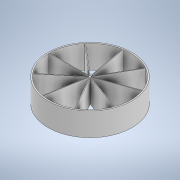
# Autodesk Inventor part: Деталь1
Saved by Autodesk Inventor 2022 (Build 260153000, 153)
## iProperties
Created: 2023-03-14
Part Number: Деталь1
Material: Типовые
Document SubType Name: Modeling
Designer: lrnto01
Density: 1 g/cm^3
Appearance: По умолчанию
Author: lrnto01
Autodesk Inventor part; units mm, degrees
ref_plane "YZ Plane" through (0, 0, 0) normal (1, 0, 0) x (0, 1, 0)
ref_plane "XZ Plane" through (0, 0, 0) normal (0, 1, 0) x (-1, 0, 0)
ref_plane "XY Plane" through (0, 0, 0) normal (0, 0, 1) x (1, 0, 0)
sketch "Эскиз1" plane through (0, 0, 0) normal (0, 1, 0) x (-1, 0, 0)
  circle A0 centre (0, 0) radius 65
  line L0 (-0.2539, 1.4397) -> (-31.066, 54.8079)
  line L1 (-59.0278, -22.0164) -> (-1.1199, -0.9397)
  line L2 (-31.066, -54.8079) -> (-0.2539, -1.4397)
  line L3 (11.4319, -61.9541) -> (0.731, -1.266)
  arc A1 (62.998, 0.5) -> (48.5807, 40.1113) centre (0, 0) ccw
  arc A2 (47.9379, 40.8774) -> (11.4319, 61.9541) centre (0, 0) ccw
  arc A3 (10.4471, 62.1278) -> (-31.066, 54.8079) centre (0, 0) ccw
  arc A4 (-31.932, 54.3079) -> (-59.0278, 22.0164) centre (0, 0) ccw
  arc A5 (-59.3698, 21.0767) -> (-59.3698, -21.0767) centre (0, 0) ccw
  arc A6 (-59.0278, -22.0164) -> (-31.932, -54.3079) centre (0, 0) ccw
  arc A7 (-31.066, -54.8079) -> (10.4471, -62.1278) centre (0, 0) ccw
  arc A8 (11.4319, -61.9541) -> (47.9379, -40.8774) centre (0, 0) ccw
  arc A9 (48.5807, -40.1113) -> (62.998, -0.5) centre (0, 0) ccw
  line L4 (0.731, 1.266) -> (11.4319, 61.9541)
  line L5 (48.5807, -40.1113) -> (1.3737, -0.5)
  line L6 (62.998, 0.5) -> (1.3737, 0.5)
  line L7 (47.9379, 40.8774) -> (0.731, 1.266)
  line L8 (1.3737, 0.5) -> (48.5807, 40.1113)
  line L9 (1.3737, -0.5) -> (62.998, -0.5)
  line L10 (0.731, -1.266) -> (47.9379, -40.8774)
  line L11 (-0.2539, -1.4397) -> (10.4471, -62.1278)
  line L12 (-1.1199, -0.9397) -> (-31.932, -54.3079)
  line L13 (-59.3698, 21.0767) -> (-1.4619, 0)
  line L14 (-1.4619, 0) -> (-59.3698, -21.0767)
  line L15 (-31.932, 54.3079) -> (-1.1199, 0.9397)
  line L16 (-1.1199, 0.9397) -> (-59.0278, 22.0164)
  line L17 (10.4471, 62.1278) -> (-0.2539, 1.4397)
  point P0 (0.0314, 0.0032)
  dimension "d1" = 130
  constraints: 36 end point, 18 point on circle, 10 centre point, 9 parallel, 2 coincident, 1 horizontal
  measures "d1" diameter of A0
extrude "Выдавливание1" add sketch "Эскиз1" along normal blind 36
